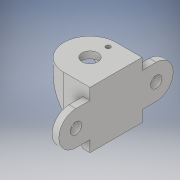
# Autodesk Inventor part: POT HOLDER
Saved by Autodesk Inventor 2019 (Build 230136000, 136)
## iProperties
Created: 2019-03-30
Part Number: POT HOLDER
Material: Generic
Document SubType Name: Modeling
Designer: torba
Density: 1 g/cm^3
Appearance: Default
Author: torba
Autodesk Inventor part; units mm, degrees
ref_plane "YZ Plane" through (0, 0, 0) normal (1, 0, 0) x (0, 1, 0)
ref_plane "XZ Plane" through (0, 0, 0) normal (0, 1, 0) x (-1, 0, 0)
sketch "Sketch2" plane through (0, 0, 0) normal (0, 1, 0) x (-1, 0, 0)
  circle A0 centre (0, 0) radius 3.5
  circle A1 centre (0, 0) radius 11.5
  line L0 (0, 0) -> (0, -8) construction
  circle A2 centre (0, -8) radius 1
  circle A3 centre (0, 0) radius 8.5 construction
  line L1 (-11.5, 0) -> (-8.5, 0) construction
  line L2 (-11.5, 11.5) -> (-8.5, 11.5) construction
  line L3 (-8.5, 11.5) -> (-8.5, -11.5) construction
  line L4 (-8.5, -11.5) -> (-11.5, -11.5) construction
  line L5 (-11.5, -11.5) -> (-11.5, 11.5)
  line L6 (-11.5, 11.5) -> (-8.5, -11.5) construction
  line L7 (-8.5, 11.5) -> (-11.5, -11.5) construction
  line L8 (-11.5, 11.5) -> (0, 11.5)
  line L9 (0, -11.5) -> (-11.5, -11.5)
  point P0 (-10, 0)
  dimension "d6" = 17
  dimension "d2" = 7
  dimension "d3" = 23
  dimension "d4" = 8
  dimension "d5" = 2
  dimension "d7" = 0
  dimension "d8" = 3
  dimension "d9" = 23
  constraints: 20 end point, 4 coincident, 3 centre point, 3 horizontal, 3 midpoint, 3 point on circle, 2 parallel, 1 horizontal alignment, 1 perpendicular, 1 tangent, 1 vertical, 2 other
  measures "d2" diameter of A0
  measures "d3" diameter of A1
  measures "d4" distance of L0.start L0.end
  measures "d5" diameter of A2
  measures "d7" distance from line of point (0, 0) L1
  measures "d8" distance of L3.end L4.end
  measures "d9" distance of L2.end L3.end
extrude "Extrusion1" add sketch "Sketch2" along normal blind 3
sketch "Sketch3" plane through (0, 0, 0) normal (0, -1, 0) x (1, 0, 0)
  line L0 (11.5, 11.5) -> (11.5, -11.5) projected
  line L1 (11.5, -11.5) -> (0, -11.5) projected
  line L2 (11.5, 11.5) -> (8.5, 11.5)
  line L3 (8.5, 11.5) -> (8.5, -11.5)
  line L4 (8.5, -11.5) -> (11.5, -11.5)
  line L5 (11.5, -11.5) -> (11.5, 11.5)
  point P0 (0, 0)
  dimension "d12" = 3
  constraints: 8 end point, 2 parallel, 1 horizontal, 1 perpendicular, 1 point on line
  measures "d12" distance of L4.end L3.end
extrude "Extrusion2" add sketch "Sketch3" along normal blind 22
sketch "Sketch4" plane through (11.5, 3, -11.5) normal (0, 0, -1) x (-1, 0, 0)
  line L0 (3, -3) -> (3, -25) projected
  line L1 (3, -25) -> (0, -25) projected
  line L2 (0, -25) -> (0, 0) projected
  line L3 (0, 0) -> (11.5, 0) projected
  line L4 (11.5, -3) -> (11.5, 0) projected
  line L5 (11.5, -3) -> (3, -3) projected
  line L6 (3, -25) -> (0, -25) projected
  line L7 (3, -25) -> (3, -3)
  line L8 (3, -3) -> (11.5, -3) projected
  line L9 (3, -3) -> (23, -3)
  line L10 (3, -3) -> (3, -25) projected
  line L11 (23, -3) -> (3, -25)
  dimension "d15" = 20
  constraints: 6 end point, 1 collinear, 1 perpendicular
  measures "d15" distance of L0.start L9.end
extrude "Extrusion3" add sketch "Sketch4" against normal up to surface (23 mm away) contours L5 L9 L11 L0
sketch "Sketch5" plane through (-11.5, 0, -11.5) normal (0, 1, 0) x (1, 0, 0)
  circle A0 centre (11.5, -11.5) radius 3.5 projected
  circle A1 centre (11.5, -3.5) radius 1 projected
  line L0 (23, -23) -> (11.5, -23) projected
  line L1 (11.5, -23) -> (0, -23) projected
  line L2 (0, -23) -> (0, -11.5) projected
  arc A2 (0, -11.5) -> (11.5, -23) centre (11.5, -11.5) ccw projected
  line L3 (23, 0) -> (23, -23) projected
  line L4 (11.5, 0) -> (23, 0) projected
  arc A3 (11.5, 0) -> (0, -11.5) centre (11.5, -11.5) ccw projected
  line L5 (0, -11.5) -> (0, 0) projected
  line L6 (0, 0) -> (11.5, 0) projected
  circle A4 centre (11.5, -11.5) radius 8.5
  dimension "d18" = 17
  constraints: 1 centre point, 1 coincident
  measures "d18" diameter of A4
extrude "Extrusion4" cut sketch "Sketch5" against normal blind 22 contours A0 | A1 A4 | A1 A4 | L1 L2 A2 | L5 L6 A3 picked at (11.4618, -3.5013) picked at (18.2153, -10.5355)
sketch "Sketch6" plane through (-11.5, 0, -11.5) normal (0, -1, 0) x (1, 0, 0)
  arc A0 (10.6086, 3.0469) -> (12.3914, 3.0469) centre (11.5, 11.5) ccw projected
  arc A1 (12.3914, 3.0469) -> (10.6086, 3.0469) centre (11.5, 11.5) ccw projected
  arc A2 (12.3914, 3.0469) -> (10.6086, 3.0469) centre (11.5, 3.5) ccw projected
  arc A3 (10.6086, 3.0469) -> (12.3914, 3.0469) centre (11.5, 3.5) ccw projected
  line L0 (23, 0) -> (11.5, 0) projected
  arc A4 (11.5, 23) -> (0, 11.5) centre (11.5, 11.5) ccw projected
  arc A5 (0, 11.5) -> (11.5, 0) centre (11.5, 11.5) ccw projected
  line L1 (11.5, 23) -> (23, 23) projected
  line L2 (23, 23) -> (23, 0) projected
  circle A6 centre (11.5, 11.5) radius 3.5 projected
extrude "Extrusion5" cut sketch "Sketch6" along normal blind 22 contours A0 A3
sketch "Sketch7" plane through (11.5, 3, 11.5) normal (1, 0, 0) x (0, 0, -1)
  line L0 (23, 0) -> (23, -25) projected
  line L1 (23, -25) -> (0, -25) projected
  line L2 (0, -25) -> (0, 0) projected
  line L3 (0, 0) -> (23, 0) projected
  line L4 (11.5, -25) -> (23, -25) projected
  line L5 (23, -15.65) -> (23, 0) projected
  line L6 (23, -25) -> (23, 0)
  line L7 (16.75, -5) -> (29.25, -5) construction
  line L8 (29.25, -5) -> (29.25, -20) construction
  line L9 (29.25, -20) -> (16.75, -20) construction
  line L10 (16.75, -20) -> (16.75, -5) construction
  line L11 (16.75, -5) -> (29.25, -20) construction
  line L12 (29.25, -5) -> (16.75, -20) construction
  circle A0 centre (29.25, -12.5) radius 2.5
  line L13 (29.25, -20) -> (23, -20)
  line L14 (23, -5) -> (29.25, -5)
  line L15 (23, -5) -> (23, -20)
  line L16 (23, -25) -> (23, -15.65) projected
  arc A1 (29.25, -20) -> (29.25, -5) centre (29.25, -12.5) ccw
  point P0 (11.5, -3)
  point P1 (23, -12.5)
  dimension "d23" = 12.5
  dimension "d24" = 15
  dimension "d25" = 5
  constraints: 20 end point, 6 midpoint, 2 centre point, 2 parallel, 2 perpendicular, 2 point on circle, 1 coincident, 1 collinear, 1 horizontal, 1 point on line, 1 vertical
  measures "d23" distance of L8.end L9.end
  measures "d24" distance of L7.end L8.end
  measures "d25" diameter of A0
extrude "Extrusion6" add sketch "Sketch7" against normal blind 3 contours L14 A1 L13 L0
ref_plane "Work Plane1" through (11.5, 3, 0) normal (0, 0, -1) x (-1, 0, 0)
mirror "Mirror1" about plane through (11.5, 3, 0) normal (0, 0, -1) of "Extrusion6"
sketch "Sketch8" plane through (-11.5, 0, -11.5) normal (0, -1, 0) x (1, 0, 0)
  arc A0 (12.3914, 3.0469) -> (10.6086, 3.0469) centre (11.5, 11.5) ccw projected
  arc A1 (10.6086, 3.0469) -> (12.3914, 3.0469) centre (11.5, 3.5) ccw projected
  arc A2 (12.3914, 3.0469) -> (10.6086, 3.0469) centre (11.5, 3.5) ccw projected
  line L0 (23, 0) -> (11.5, 0) projected
  arc A3 (11.5, 23) -> (0, 11.5) centre (11.5, 11.5) ccw projected
  arc A4 (0, 11.5) -> (11.5, 0) centre (11.5, 11.5) ccw projected
  line L1 (11.5, 23) -> (23, 23) projected
  line L2 (23, 23) -> (23, 0) projected
  circle A5 centre (11.5, 11.5) radius 3.5 projected
  line L3 (23, 23) -> (23, 0) projected
  line L4 (0, 3) -> (12.366, 3)
  line L5 (23, 3) -> (23, 20)
  line L6 (11.5, 20) -> (0, 20)
  line L7 (0, 20) -> (0, 3)
  line L8 (0, 3) -> (23, 20) construction
  line L9 (23, 3) -> (0, 20) construction
  line L10 (11.5, 20) -> (11.5, 3)
  dimension "d28" = 11.5
  constraints: 14 end point, 3 parallel, 3 tangent, 2 midpoint, 2 point on line, 1 horizontal, 1 perpendicular, 1 point on circle
  measures "d28" distance between parallel lines of L10 L3
extrude "Extrusion7" cut sketch "Sketch8" along normal up to next contours L10 A5 A2 A0 | A0 A1 L4 A4 A3 L6 | L10 L4 A1 A2 | A3 L7 L6 | L10 A5 | A4 L4 L7 picked at (9.8069, 5.387) picked at (11.4251, 3.9914) picked at (10.168, 10.6267)
body "Solid1"
